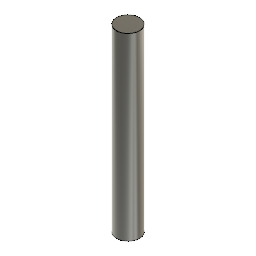
Arm Dowel Pin (Autodesk Fusion 360 design; units mm, degrees)
Autodesk Fusion 360 part; units mm, degrees
sketch "Sketch1" plane through (0, 0, 0) normal (0, 0, 1) x (1, 0, 0)
  circle A0 centre (0, 0) radius 3.74
  dimension "d3" = 7.48
  constraint coincident A0.centre origin
  measures "d3" diameter of A0
extrude "Extrude1" add sketch "Sketch1" along normal blind 58
equation "dowel_pin_radius = 3.74 mm"
equation "length = 58 mm"
equation "d3 = dowel_pin_radius * 2"
equation "d4 = length"
